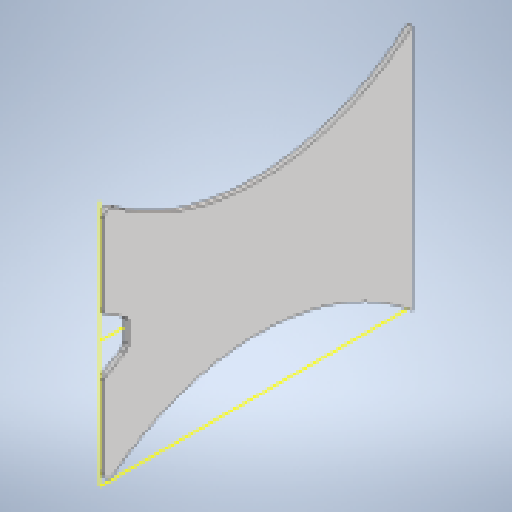
# Autodesk Inventor part: грань тела
Saved by Autodesk Inventor 2023.1 (Build 271208000, 208)
## iProperties
Created: 2024-11-21
Part Number: грань тела
Material: Типовые
Document SubType Name: Modeling
Designer: DELL
Density: 1 g/cm^3
Appearance: По умолчанию
Author: DELL
Autodesk Inventor part; units mm, degrees
ref_plane "YZ Plane" through (0, 0, 0) normal (1, 0, 0) x (0, 1, 0)
ref_plane "XZ Plane" through (0, 0, 0) normal (0, 1, 0) x (-1, 0, 0)
ref_plane "XY Plane" through (0, 0, 0) normal (0, 0, 1) x (1, 0, 0)
sketch "Эскиз1" plane through (0, 0, 0) normal (0, 0, 1) x (1, 0, 0)
  line L0 (2, -100) -> (-2, -100)
  line L1 (-2, -100) -> (-2, 100)
  line L2 (-2, 100) -> (2, 100)
  line L3 (2, 100) -> (2, -100)
  line L4 (2, -100) -> (-2, 100) construction
  line L5 (-2, -100) -> (2, 100) construction
  point P0 (0, 0)
  dimension "d0" = 4
  dimension "d1" = 200
  constraints: 12 end point, 2 midpoint, 2 parallel, 1 horizontal, 1 perpendicular
  measures "d0" distance of L1.end L2.end
  measures "d1" distance of L0.end L1.end
extrude "Выдавливание1" add sketch "Эскиз1" along normal blind 250
sketch "Эскиз2" plane through (-2, -100, 0) normal (-1, 0, 0) x (0, 0, 1)
  line L0 (250, 200) -> (250, 0) projected
  line L1 (0, 0) -> (250, 0) projected
  line L2 (0, 102) -> (250, 102) projected
  point P0 (0, 100)
sketch "Эскиз3" plane through (2, -100, 0) normal (1, 0, 0) x (0, 0, -1)
  line L0 (0, 0) -> (0, 200) construction
  line L1 (0, 200) -> (-250, 200) construction
  line L2 (-250, 0) -> (-250, 200) construction
  line L3 (0, 0) -> (-250, 0) construction
  line L4 (-250, 200) -> (-250, 0) construction
  line L5 (-250, 0) -> (0, 200) construction
  line L6 (0, 100) -> (-250, 100) construction
  line L7 (0, 200) -> (-250, 200) projected
  arc A0 (-250, 200) -> (0, 200) centre (-125, 344.0414) ccw
  arc A1 (0, 0) -> (-250, 0) centre (-125, -144.0414) ccw
  line L8 (-250, 0) -> (0, 0)
  constraints: 6 end point, 4 point on circle, 2 centre point, 1 midpoint, 1 perpendicular, 1 symmetric about line, 1 other
extrude "Выдавливание2" cut sketch "Эскиз3" against normal blind 4
fillet "Сопряжение1" radius 5 1 edges at (0, 100, 250)
fillet "Сопряжение2" radius 5 1 edges at (0, -100, 250)
sketch "Эскиз4" plane through (-2, -100, 0) normal (-1, 0, 0) x (0, 0, 1)
  arc A0 (250, 189.4287) -> (241.9343, 193.3786) centre (245, 189.4287) ccw projected
  arc A1 (241.9343, 6.6214) -> (250, 10.5713) centre (245, 10.5713) ccw projected
  line L0 (248.5, 78.2507) -> (232.9146, 87.249)
  line L1 (230.4146, 91.5791) -> (230.4146, 108.4209)
  line L2 (232.9146, 112.751) -> (248.5, 121.7493)
  arc A2 (232.9146, 112.751) -> (230.4146, 108.4209) centre (235.4146, 108.4209) ccw
  arc A3 (230.4146, 91.5791) -> (232.9146, 87.249) centre (235.4146, 91.5791) ccw
  arc A4 (248.5, 121.7493) -> (250, 124.3473) centre (247, 124.3473) ccw
  arc A5 (250, 75.6527) -> (248.5, 78.2507) centre (247, 75.6527) ccw
  line L3 (250, 124.3473) -> (250, 75.6527)
  line L4 (250, 10.5713) -> (250, 189.4287) projected
  point P0 (0, 100)
  point P1 (250, 100)
  point P2 (250, 77.3847)
  point P3 (230.4146, 88.6924)
  point P4 (230.4146, 111.3076)
  point P5 (250, 122.6153)
  dimension "d8" = 5
  dimension "d9" = 3
  constraints: 8 end point, 8 point on circle, 6 point on line, 6 tangent, 4 centre point, 2 equal radius, 1 collinear, 6 other
  measures "d8" radius of A2
  measures "d9" radius of A4
extrude "Выдавливание3" cut sketch "Эскиз4" against normal blind 4
